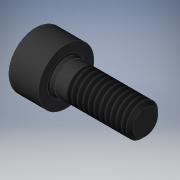
# Autodesk Inventor part: M4x10_p3
Saved by Autodesk Inventor 2019 (Build 230136000, 136)
## iProperties
Created: 2024-03-05
Part Number: M4x10_p3
Material: Generic
Catalog Web Link: www.cadenas.de
Description: MBRDC, MBRDAC_part3-Pulleys for Round Belts - Clemping Type - Trapezoid Groove
Vendor: MISUMI
Document SubType Name: Modeling
Designer: psAdmin
Manufacturer: MISUMI
Mass: 0.256179 g
Surface Area: 3.08224 cm^2
Volume: 0.256179 cm^3
Density: 1 g/cm^3
Appearance: PSOLRGB-175-175-175
Category: PARTsolutions
Company: MISUMI
Title: M4x10
Author: Cadenas PARTsolutions
Comments: Pulleys for Round Belts - Clemping Type - Trapezoid Groove
PSOL_IDENT_0: {$CADENAS_DATA/23d-libs/misumi/metric/52_belts_pulleys/mbrdc/mbrdc_part3.prj},167 {VTYP=3D},{NB=M4x1
PSOL_IDENT_1: 0_p3},{LINA=M4x10},{NN=MBRDC, MBRDAC_part3},{DATE=06.06.2021 23:11:25},{GEOMDATE=10.06.2016 02:58:32
PSOL_IDENT_2: },{VERSION=},{LINEID=390},{WBVAR=},{WBNUMERIC=}  {NB=M4x10_p3},{LINA=M4x10},{KT=DUMMY},{PN=M4x10},{D=
PSOL_IDENT_3: 4.000},{D3=3.141},{P=0.700},{L=10.000},{S=3.000},{HM=10.000},{DK=7.000},{DA=4.700},{DS=4.000},{E=3.4
PSOL_IDENT_4: 40},{K=4.000},{R=0.200},{T=2.000},{V=0.400},{DW=6.530},{W=1.400},{LF=0.600},{LG=2.100},{FORM=1.000}
NB: M4x10_p3
NN: MBRDC, MBRDAC_part3
NT: Pulleys for Round Belts - Clemping Type - Trapezoid Groove
NBSYN: $PN._p3
LINA: M4x10
CATALOG: Misumi
PN: M4x10
D: 4
D3: 3.141
P: 0.7
L: 10
S: 3
HM: 10
DK: 7
DA: 4.7
DS: 4
E: 3.44
K: 4
R: 0.2
T: 2
V: 0.4
DW: 6.53
W: 1.4
LF: 0.6
LG: 2.1
FORM: 1
SUPPLIER: MISUMI
ARTICLENO: M4x10_p3
BOMINFO: M4x10
CREATOR: CADENAS GmbH
Autodesk Inventor part; units mm, degrees
sketch "Skizze_2" plane through (0, 0, 0) normal (0, 0, 1) x (1, 0, 0)
  line L0 (10, 0) -> (-7, 0)
  line L1 (-0.534, 0) -> (-1.4, 1.5)
  line L2 (-1.4, 1.5) -> (-3.78, 1.5)
  line L3 (-3.78, 1.5) -> (-4, 1.72)
  line L4 (-4, 1.72) -> (-4, 3.1)
  arc A0 (-3.6, 3.5) -> (-4, 3.1) centre (-3.6, 3.1) ccw
  line L5 (-3.6, 3.5) -> (0, 3.5)
  line L6 (0, 3.5) -> (0, 2.35)
  arc A1 (0, 2.35) -> (0.1298, 2.1627) centre (0.2, 2.35) ccw
  line L7 (0.1298, 2.1627) -> (0.5298, 2.0127)
  arc A2 (0.5298, 2.0127) -> (0.6, 2) centre (0.6, 2.2) ccw
  line L8 (0.6, 2) -> (9.5705, 2)
  line L9 (9.5705, 2) -> (10, 1.5705)
  line L10 (10, 1.5705) -> (10, 0)
  line L11 (10, 0) -> (-0.534, 0)
  constraints: 24 end point, 6 point on circle, 3 centre point
revolve "Revolution1" add sketch "Skizze_2" angle 360 about axis through (10, 0, 0) along (1, 0, 0)
thread "Thread1" size "M4x0.7" class "6g" standard "ISO Metric profile" length 7.4705
sketch "Skizze_1" plane through (-1.4, 0, 0) normal (1, 0, 0) x (0, 0, -1)
  line L0 (-1.5, -0.866) -> (0, -1.7321)
  line L1 (0, -1.7321) -> (1.5, -0.866)
  line L2 (1.5, -0.866) -> (1.5, 0.866)
  line L3 (1.5, 0.866) -> (0, 1.7321)
  line L4 (0, 1.7321) -> (-1.5, 0.866)
  line L5 (-1.5, 0.866) -> (-1.5, -0.866)
  constraints: 12 end point
extrude "Extrusion1" cut sketch "Skizze_1" against normal blind 4
ref_plane "IP1_XY" through (0, 0, 0) normal (1, 0, 0) x (0, 0, -1)
ref_plane "IP1_YZ" through (0, 0, 0) normal (0, 0, -1) x (0, 1, 0)
ref_plane "IP1_ZX" through (0, 0, 0) normal (0, 1, 0) x (1, 0, 0)
ref_plane "IP2_XY" through (-4, 0, 0) normal (1, 0, 0) x (0, 0, -1)
ref_plane "IP2_YZ" through (-4, 0, 0) normal (0, 0, -1) x (0, 1, 0)
ref_plane "IP2_ZX" through (-4, 0, 0) normal (0, 1, 0) x (1, 0, 0)
ref_plane "IP3_XY" through (10, 0, 0) normal (1, 0, 0) x (0, 0, -1)
ref_plane "IP3_YZ" through (10, 0, 0) normal (0, 0, -1) x (0, 1, 0)
ref_plane "IP3_ZX" through (10, 0, 0) normal (0, 1, 0) x (1, 0, 0)
body "Solid1"
